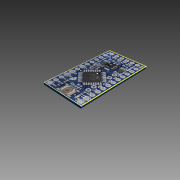
# Autodesk Inventor part: ArduinoProMini
Saved by Autodesk Inventor 2014 (Build 180170000, 170)
## iProperties
Created: 2013-11-03
Part Number: ArduinoProMini
Material: Generic
Document SubType Name: Modeling
Designer: blacki
Density: 1 g/cm^3
Appearance: Arduino
Author: blacki
Autodesk Inventor part; units mm, degrees
ref_plane "YZ Plane" through (0, 0, 0) normal (1, 0, 0) x (0, 1, 0)
ref_plane "XZ Plane" through (0, 0, 0) normal (0, 1, 0) x (-1, 0, 0)
ref_plane "XY Plane" through (0, 0, 0) normal (0, 0, 1) x (1, 0, 0)
sketch "Sketch1" plane through (0, 0, 0) normal (0, 0, 1) x (1, 0, 0)
  line L0 (-9, 16.5) -> (9, 16.5)
  line L1 (9, 16.5) -> (9, -16.5)
  line L2 (9, -16.5) -> (-9, -16.5)
  line L3 (-9, -16.5) -> (-9, 16.5)
  line L4 (-9, 16.5) -> (9, -16.5) construction
  line L5 (9, 16.5) -> (-9, -16.5) construction
  point P0 (0, 0)
  dimension "d0" = 18
  dimension "d1" = 33
  constraints: 12 end point, 2 midpoint, 2 parallel, 1 horizontal, 1 perpendicular
  measures "d0" distance of L1.end L2.end
  measures "d1" distance of L0.end L1.end
extrude "Extrusion1" add sketch "Sketch1" along normal blind 1
sketch "Sketch2" plane through (0, 0, 1) normal (0, 0, 1) x (1, 0, 0)
  line L0 (9, 16.5) -> (-9, 16.5) projected
  line L1 (9, -16.5) -> (9, 16.5) projected
  line L2 (-9, 16.5) -> (9.2657, 16.5) construction
  line L3 (9.2657, 16.5) -> (9.2657, -16.5211) construction
  line L4 (9.2657, -16.5211) -> (-9, -16.5211) construction
  line L5 (-9, -16.5211) -> (-9, 16.5) construction
  point P0 (0, 0)
  constraints: 2 other
body "Solid1"
